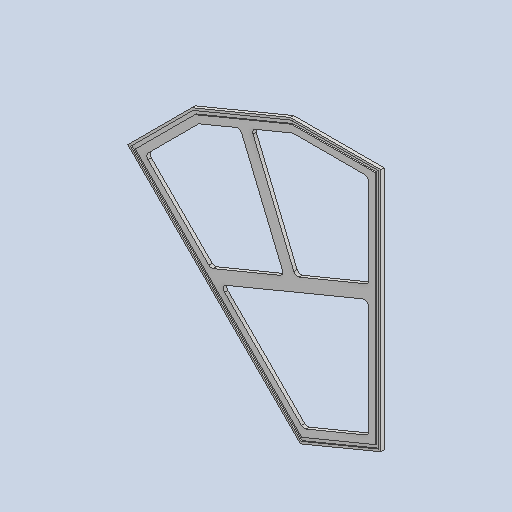
# Autodesk Inventor part: ДМФ 01 51 Внешняя рамка v2.0
Saved by Autodesk Inventor 2025 (Build 290162010, 162A)
## iProperties
Created: 2024-05-05
Part Number: ДМФ 01 51 Внешняя рамка v2.0
Material: Generic
Document SubType Name: Modeling
Designer: pokla
Density: 1 g/cm^3
Appearance: Default
Author: pokla
Autodesk Inventor part; units mm, degrees
ref_plane "YZ Plane" through (0, 0, 0) normal (1, 0, 0) x (0, 1, 0)
ref_plane "XZ Plane" through (0, 0, 0) normal (0, 1, 0) x (-1, 0, 0)
ref_plane "XY Plane" through (0, 0, 0) normal (0, 0, 1) x (1, 0, 0)
sketch "Sketch1" plane through (0, 0, 0) normal (0, 0, 1) x (1, 0, 0)
  line L0 (0, 277.6336) -> (196.3166, 196.3166) construction
  line L1 (196.3166, 196.3166) -> (277.6336, 0) construction
  line L2 (277.6336, 0) -> (196.3166, -196.3166) construction
  line L3 (196.3166, -196.3166) -> (0, -277.6336) construction
  line L4 (0, -277.6336) -> (-196.3166, -196.3166) construction
  line L5 (-196.3166, -196.3166) -> (-277.6336, 0) construction
  line L6 (-277.6336, 0) -> (-196.3166, 196.3166) construction
  line L7 (-196.3166, 196.3166) -> (0, 277.6336)
  line L8 (-196.3166, 196.3166) -> (0, 277.6336)
  line L9 (-461.2666, 773.8898) -> (-221.0579, 873.3874)
  line L10 (-98.1583, 236.9751) -> (-341.1623, 823.6386) construction
  line L11 (-221.0579, 873.3874) -> (0, 873.3874)
  line L12 (0, 873.3874) -> (0, 277.6336)
  line L13 (-461.2666, 773.8898) -> (-617.5782, 617.5782)
  line L14 (-617.5782, 617.5782) -> (-196.3166, 196.3166)
  point P0 (0, 0)
  point P1 (0, 0)
  dimension "d0" = 513
  dimension "d2" = 260
  dimension "d3" = 635
  constraints: 30 end point, 2 midpoint, 1 coincident, 1 horizontal, 1 parallel, 1 perpendicular, 1 symmetric about line, 1 vertical, 1 vertical alignment, 17 other
  measures "d0" distance between parallel lines of L5 L1
  measures "d2" distance of L9.start L9.end
  measures "d3" distance of L10.end L10.start
extrude "Extrusion1" add sketch "Sketch1" along normal mid plane 8
sketch "Sketch2" plane through (0, 0, 4) normal (0, 0, 1) x (1, 0, 0)
  line L0 (-221.0579, 873.3874) -> (-461.2666, 773.8898) projected
  line L1 (-461.2666, 773.8898) -> (-617.5782, 617.5782) projected
  line L2 (-236.3886, 531.4957) -> (-415.0608, 457.4872)
  line L3 (-196.3166, 196.3166) -> (0, 277.6336) projected
  line L4 (-98.1583, 236.9751) -> (-341.1623, 823.6386) construction
  line L5 (-617.5782, 617.5782) -> (-196.3166, 196.3166) projected
  line L6 (-415.0608, 457.4872) -> (-575.1518, 617.5782)
  line L7 (-575.1518, 617.5782) -> (-444.273, 748.457)
  line L8 (-444.273, 748.457) -> (-343.54, 790.182)
  line L9 (-236.3886, 531.4957) -> (-343.54, 790.182)
  line L10 (-208.6722, 542.9762) -> (-30, 616.9847)
  line L11 (-30, 616.9847) -> (-30, 843.3874)
  line L12 (-30, 843.3874) -> (-215.0906, 843.3874)
  line L13 (-215.0906, 843.3874) -> (-315.8236, 801.6625)
  line L14 (-208.6722, 542.9762) -> (-315.8236, 801.6625)
  line L15 (0, 277.6336) -> (0, 873.3874) projected
  line L16 (-415.0608, 457.4872) -> (-30, 616.9847) construction
  line L17 (-392.0998, 434.5262) -> (-30, 584.5129)
  line L18 (-189.2776, 231.704) -> (-30, 297.679)
  line L19 (-30, 297.679) -> (-30, 584.5129)
  line L20 (-189.2776, 231.704) -> (-392.0998, 434.5262)
  point P0 (0, 0)
  dimension "d11" = 30
  dimension "d12" = 280
  dimension "d13" = 30
  dimension "d14" = 30
  dimension "d15" = 15
  dimension "d21" = 30
  dimension "d22" = 30
  dimension "d23" = 30
  dimension "d24" = 30
  constraints: 32 end point, 5 parallel, 5 symmetric about line, 2 midpoint, 1 collinear
  measures "d11" distance between parallel lines of L5 L6
  measures "d12" distance between parallel lines of L8 L2
  measures "d13" distance between parallel lines of L0 L8
  measures "d14" distance between parallel lines of L1 L7
  measures "d15" distance between parallel lines of L9 L4
  measures "d21" distance between parallel lines of L16 L17
  measures "d22" distance between parallel lines of L5 L20
  measures "d23" distance between parallel lines of L19 L15
  measures "d24" distance between parallel lines of L18 L3
extrude "Extrusion2" cut sketch "Sketch2" against normal up to surface (8 mm away)
fillet "Fillet1" radius 10 12 edges at (-575.1518, 617.5782, 0) (-343.54, 790.182, 0) (-236.3886, 531.4957, 0) (-415.0608, 457.4872, 0) (-315.8236, 801.6625, 0) (-30, 843.3874, 0) (-30, 616.9847, 0) (-208.6722, 542.9762, 0) (-392.0998, 434.5262, 0) (-30, 584.5129, 0) (-30, 297.679, 0) (-189.2776, 231.704, 0)
sketch "Sketch4" plane through (0, 0, 4) normal (0, 0, 1) x (1, 0, 0)
  line L0 (-221.0579, 873.3874) -> (-461.2666, 773.8898) projected
  line L1 (0, 873.3874) -> (-221.0579, 873.3874) projected
  line L2 (-461.2666, 773.8898) -> (-617.5782, 617.5782) projected
  line L3 (-617.5782, 617.5782) -> (-196.3166, 196.3166) projected
  line L4 (-196.3166, 196.3166) -> (0, 277.6336) projected
  line L5 (0, 277.6336) -> (0, 873.3874) projected
  line L6 (-458.4343, 769.651) -> (-220.0634, 868.3874)
  line L7 (-220.0634, 868.3874) -> (-5, 868.3874)
  line L8 (-5, 868.3874) -> (-5, 280.9745)
  line L9 (-5, 280.9745) -> (-195.1434, 202.2145)
  line L10 (-195.1434, 202.2145) -> (-610.5071, 617.5782)
  line L11 (-610.5071, 617.5782) -> (-458.4343, 769.651)
  line L12 (-218.4721, 860.3874) -> (-453.9027, 762.8689)
  line L13 (-453.9027, 762.8689) -> (-599.1934, 617.5782)
  line L14 (-599.1934, 617.5782) -> (-193.2664, 211.6511)
  line L15 (-193.2664, 211.6511) -> (-13, 286.3199)
  line L16 (-13, 286.3199) -> (-13, 860.3874)
  line L17 (-13, 860.3874) -> (-218.4721, 860.3874)
  point P0 (0, 0)
  dimension "d26" = 5
  dimension "d27" = 8
  constraints: 24 end point, 10 other
  measures "d26" distance between parallel lines of L0 L6
  measures "d27" distance between parallel lines of L6 L12
extrude "Extrusion3" cut sketch "Sketch4" against normal blind 3 contours L6 L7 L8 L9 L10 L11
fillet "Fillet3" radius 16 2 edges at (-220.0634, 868.3874, 2.5) (-458.4343, 769.651, 2.5)
fillet "Fillet4" radius 8 2 edges at (-453.9027, 762.8689, 2.5) (-218.4721, 860.3874, 2.5)
equation "\"d0\" = Барабан_габарит_по_кассетам"
equation "\"d2\" = Кассета_длина_грани"
equation "\"d3\" = Кассета_высота"
equation "\"d11\" = d13"
equation "\"d14\" = d13"
equation "\"d15\" = 0.5 * d13"
equation "\"d21\" = d13"
equation "\"d22\" = d13"
equation "\"d23\" = d13"
equation "\"d24\" = d13"
equation "\"Барабан_габарит_по_кассетам\" = 513"
equation "\"Кассета_длина_грани\" = 260"
equation "\"Кассета_высота\" = 635"
body "Solid1"
